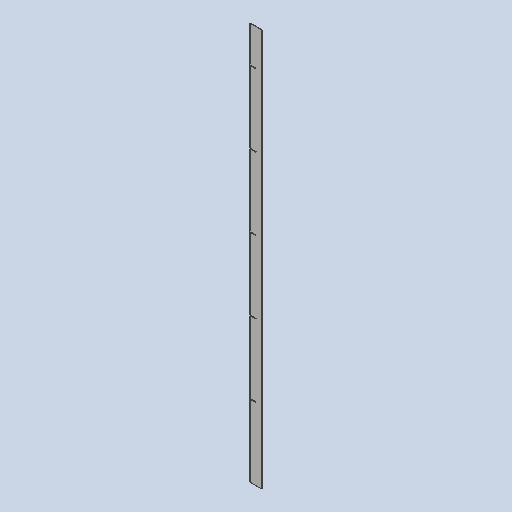
# Autodesk Inventor part: BSH 034 stringer board 2
Saved by Autodesk Inventor 2025 (Build 290162010, 162A)
## iProperties
Created: 2024-07-23
Part Number: BSH 034 stringer board 2
Material: 09g2s
Document SubType Name: Sheet Metal
Designer: pokla
Density: 7.85 g/cm^3
Sheet Metal Rule: AISI304 3mm Die 32
Sheet Metal Width: 80,639 mm
Sheet Metal Length: 2751,500 mm
Sheet Metal Area: 221879,387 mm^2
Appearance: Default
Mass: 5209.69 g
Surface Area: 4606.69 cm^2
Volume: 663.655 cm^3
Flat Pattern Width: 8.06394 cm
Flat Pattern Length: 275.15 cm
Flat Pattern Area: 2218.79 cm^2
Stock Number: БШК 034 стрингер борт 2
Author: admin
Autodesk Inventor part; units mm, degrees
ref_plane "YZ Plane" through (0, 0, 0) normal (1, 0, 0) x (0, 1, 0)
ref_plane "XZ Plane" through (0, 0, 0) normal (0, 1, 0) x (-1, 0, 0)
ref_plane "XY Plane" through (0, 0, 0) normal (0, 0, 1) x (1, 0, 0)
sketch "Sketch6" plane through (0, 0, 0) normal (0, 1, 0) x (-1, 0, 0)
  line L0 (0, 0) -> (-80.6394, 0)
  line L1 (-80.6394, 0) -> (-80.6394, 2751.5)
  line L2 (-80.6394, 2751.5) -> (0, 2751.5)
  line L3 (0, 2751.5) -> (0, 0)
  dimension "d26" = 80.6394
  dimension "d27" = 2751.5
  measures "d26" distance of L1.end L2.end
  measures "d27" distance of L0.end L1.end
extrude "Plate4" add sketch "Sketch6" along normal blind 3
sketch "Sketch7" plane through (0, 0, 0) normal (0, -1, 0) x (1, 0, 0)
  line L0 (0, 2751.5) -> (80.6394, 2751.5) projected
  line L1 (0, 0) -> (0, 2751.5) projected
  line L2 (80.6394, 0) -> (0, 0) projected
  line L3 (80.6394, 2751.5) -> (80.6394, 0) projected
  line L4 (0, 501.7) -> (41.3197, 501.7)
  line L5 (41.3197, 501.7) -> (41.3197, 498.5)
  line L6 (41.3197, 498.5) -> (0, 498.5)
  line L7 (0, 498.5) -> (0, 501.7)
  point P0 (0, 498.5)
  point P1 (0, 200)
  point P2 (46.4173, 200)
  point P3 (0, 498.5)
  dimension "d29" = 41.3197
  dimension "d30" = 3.2
  dimension "d31" = 498.5
  constraints: 8 end point, 2 parallel, 1 horizontal, 1 perpendicular, 1 point on line
  measures "d29" distance of L5.end L6.end
  measures "d30" distance of L4.end L5.end
  measures "d31" distance between parallel lines of L2 L6
extrude "Extrusion2" cut sketch "Sketch7" against normal through all contours L4 L5 L6 L1
pattern_linear "Rectangular Pattern1" count 5 spacing 500 along (0, 0, 1) of "Extrusion2"
equation "\"d26\" = Stringer2_deep"
equation "\"d28\" = Thickness"
equation "\"BendReliefWidth\" = Thickness"
equation "\"BendReliefDepth\" = 0.5 * Thickness"
equation "\"CornerReliefSize\" = 4 * Thickness"
equation "\"MinimumRemnant\" = 2 * Thickness"
equation "\"TransitionRadius\" = BendRadius"
equation "\"JacobiRadiusSize\" = BendRadius"
equation "\"GapSize\" = Thickness"
equation "\"Stringer2_deep\" = 80.639428"
equation "\"Thickness\" = 3"
equation "\"BendRadius\" = 5"
body "Solid2"
